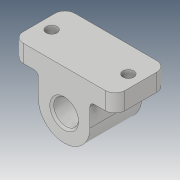
# Autodesk Inventor part: shaftMount
Saved by Autodesk Inventor 2018 (Build 220112000, 112)
## iProperties
Created: 2020-02-27
Part Number: shaftMount
Material: Generic
Document SubType Name: Modeling
Designer: anirudh
Density: 1 g/cm^3
Appearance: Default
Author: anirudh
Autodesk Inventor part; units mm, degrees
ref_plane "YZ Plane" through (0, 0, 0) normal (1, 0, 0) x (0, 1, 0)
ref_plane "XZ Plane" through (0, 0, 0) normal (0, 1, 0) x (-1, 0, 0)
ref_plane "XY Plane" through (0, 0, 0) normal (0, 0, 1) x (1, 0, 0)
sketch "Sketch1" plane through (0, 0, 0) normal (0, 1, 0) x (-1, 0, 0)
  circle A0 centre (-92.5739, -114.0841) radius 1.75
  line L0 (-104.8331, -105.8291) -> (-88.5698, -105.8291)
  line L1 (-88.5698, -105.8291) -> (-88.5698, -122.3391)
  line L2 (-88.5698, -122.3391) -> (-104.8331, -122.3391)
  line L3 (-104.8331, -105.8291) -> (-121.0891, -105.8291)
  line L4 (-121.0891, -105.8291) -> (-121.0891, -122.3391)
  line L5 (-121.0891, -122.3391) -> (-104.8331, -122.3391)
  circle A1 centre (-117.0886, -114.0841) radius 1.75
  point P0 (0, 0)
  point P1 (0, 0)
  constraints: 12 end point, 2 centre point, 2 perpendicular, 2 point on line
extrude "Extrusion1" add sketch "Sketch1" along normal blind 5.588
sketch "Sketch2" plane through (88.5698, 0, -105.8291) normal (0, 0, 1) x (1, 0, 0)
  line L0 (0, 5.588) -> (32.5193, 5.588) projected
  line L1 (0, 5.588) -> (32.5193, 5.588)
  arc A0 (8.0046, -7.239) -> (24.5146, -7.239) centre (16.2596, -7.239) ccw
  line L2 (8.0046, -7.239) -> (8.0046, 0)
  line L3 (0, 0) -> (32.5193, 0) projected
  line L4 (8.0046, 0) -> (24.5146, 0)
  line L5 (24.5146, 0) -> (24.5146, -7.239)
  circle A1 centre (16.2596, -7.2898) radius 3.9688
  point P0 (-88.5698, 0)
  dimension "d14" = 7.9375
  constraints: 8 end point, 2 centre point, 2 horizontal, 2 point on circle, 1 perpendicular, 1 point on line, 1 vertical
  measures "d14" diameter of A1
fillet "Fillet2" radius 3.175 4 edges at (88.5698, 2.794, -122.3391) (88.5698, 2.794, -105.8291) (121.0891, 2.794, -122.3391) (121.0891, 2.794, -105.8291)
extrude "Extrusion3" add sketch "Sketch2" against normal blind 16.51
fillet "Fillet3" radius 1.27 2 edges at (96.5744, 0, -114.0841) (113.0844, 0, -114.0841)
chamfer "Chamfer2" distance 0.635 angle 45 2 edges at (100.8607, -7.2898, -105.8291) (100.8607, -7.2898, -122.3391)
body "Solid1"
